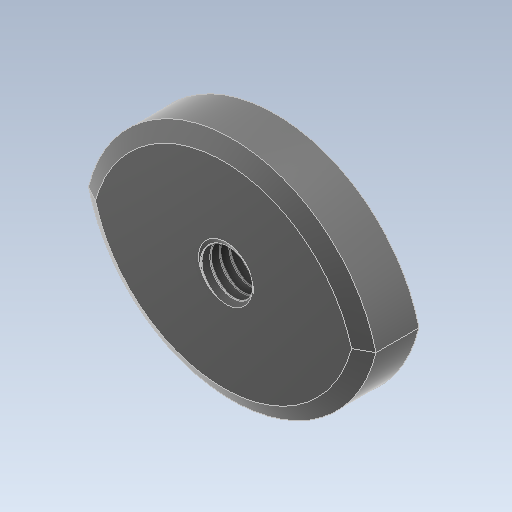
# Autodesk Inventor part: BobbinGuidePlate
Saved by Autodesk Inventor 2021 (Build 250183000, 183)
## iProperties
Created: 2020-03-09
Part Number: BobbinGuidePlate
Material: Generic
Document SubType Name: Modeling
Designer: elmar
Density: 1 g/cm^3
Appearance: Smooth - Black
Author: elmar
Autodesk Inventor part; units mm, degrees
ref_plane "YZ Plane" through (0, 0, 0) normal (1, 0, 0) x (0, 1, 0)
ref_plane "XZ Plane" through (0, 0, 0) normal (0, 1, 0) x (-1, 0, 0)
ref_plane "XY Plane" through (0, 0, 0) normal (0, 0, 1) x (1, 0, 0)
sketch "Sketch1" plane through (0, 0, 0) normal (0, 0, 1) x (1, 0, 0)
  circle A0 centre (0, 0) radius 15
  circle A1 centre (0, 0) radius 19
  arc A2 (19, 0) -> (-19, 0) centre (0, -4.5333) ccw
  arc A3 (-19, 0) -> (19, 0) centre (0, 4.5333) ccw
  line L0 (-26.6, 0) -> (26.6, 0) projected
  point P0 (0, 15)
  point P1 (0, -15)
  dimension "CarriageGuidePlateDiameter" = 30
  dimension "d70" = 38
  constraints: 6 point on circle, 4 centre point, 2 coincident, 2 point on line, 2 tangent
  measures "CarriageGuidePlateDiameter" diameter of A0
  measures "d70" diameter of A1
extrude "Extrusion1" add sketch "Sketch1" along normal blind 8 contours L0 A0 | L0 A3 A0 | A0 A2 L0 | A0 L0 | A0 L0 A2 | A3 L0 A0
sketch "Sketch2" plane through (0, 0, 0) normal (0, 0, -1) x (-1, 0, 0)
  point P0 (0, 0)
hole "Hole1" at (0, 0, 0) direction (0, 0, 1) diameter 8 end through all
thread "Thread1" size "M8x1.25" class "6H" standard "ANSI Metric M Profile" full length
sketch "Sketch8" plane through (0, 0, 0) normal (1, 0, 0) x (0, 1, 0)
  line L0 (4, 0) -> (4, 8)
  line L1 (4, 8) -> (3.0732, 8)
  line L2 (3.0732, 8) -> (3.0732, 0)
  line L3 (3.0732, 0) -> (4, 0)
  line L4 (0, -1.6) -> (0, 9.6) projected
  constraints: 8 end point
revolve "Revolution3" add sketch "Sketch8" angle 360 about axis through (0, 0, 0) along (0, 0, 1) separate body
sketch "Sketch7" plane through (0, 4, 0) normal (-1, 0, 0) x (0, 0, 1)
  line L0 (-0.7293, -0.0634) -> (-0.6251, -0.0634) construction
  line L1 (0.1041, -0.8638) -> (-0.0001, -1.0639) construction
  line L2 (-1.2501, -1.0639) -> (-1.3543, -0.8638) construction
  line L3 (-0.5209, -0.0634) -> (-0.6251, 0.1367) construction
  line L4 (-0.6251, 0.1367) -> (-0.7293, -0.0634) construction
  line L5 (-1.2501, -1.0639) -> (-1.1459, -0.8638) construction
  line L6 (-0.5209, -0.0634) -> (-0.1043, -0.8638)
  line L7 (-1.3543, -0.8638) -> (-1.1459, -0.8638) construction
  arc A0 (-1.3543, -0.8638) -> (-1.2501, -0.927) centre (-1.2501, -0.8096) ccw construction
  line L8 (0.1041, -0.8638) -> (-0.1043, -0.8638) construction
  line L9 (-1.2501, -1.0639) -> (-1.2501, -0.8638) construction
  line L10 (-0.0001, -1.0639) -> (-0.0001, -0.8638) construction
  line L11 (-0.6251, 0.1367) -> (-0.6251, -0.0002) construction
  line L12 (-1.2501, -0.927) -> (-0.0001, -0.927)
  arc A1 (-1.2501, -0.927) -> (-1.1459, -0.8638) centre (-1.2501, -0.8096) ccw
  line L13 (-0.1043, -0.8638) -> (-0.0001, -1.0639) construction
  line L14 (-1.1459, -0.8638) -> (-0.7293, -0.0634)
  line L15 (-0.0001, -0.0002) -> (-0.0001, 0.0177)
  line L16 (-0.0001, 0.0177) -> (-0.0001, -0.0002)
  line L17 (-0.0001, -0.0002) -> (0.0334, -0.0002)
  arc A2 (-0.1043, -0.8638) -> (-0.0001, -0.927) centre (-0.0001, -0.8096) ccw
  arc A3 (-0.0001, -0.927) -> (0.1041, -0.8638) centre (-0.0001, -0.8096) ccw construction
  arc A4 (-0.6251, -0.0002) -> (-0.7293, -0.0634) centre (-0.6251, -0.1176) ccw
  arc A5 (-0.5209, -0.0634) -> (-0.6251, -0.0002) centre (-0.6251, -0.1176) ccw
  line L18 (-0.6251, -0.0002) -> (-0.6251, -0.0634) construction
  line L19 (-0.6251, -0.0634) -> (-0.5209, -0.0634) construction
  dimension "d49" = 55
  dimension "d50" = 0.2001
  dimension "d51" = 0.2001
  dimension "Sketch7_ThreadOffset" = 0
  dimension "Sketch7_MajorRadius" = 0.9268
  dimension "d54" = 1.25
  dimension "Sketch7_MinorRadius" = 0
  constraints: 40 end point, 12 point on circle, 10 parallel, 8 tangent, 6 centre point, 6 collinear, 2 midpoint, 2 point on line, 1 horizontal, 1 perpendicular, 3 other
  measures "d49" angle of L6 L14
  measures "d50" distance of L3.end L0.end
  measures "d51" distance of L1.end L10.end
  measures "Sketch7_ThreadOffset" distance between parallel lines of L15 L10
  measures "Sketch7_MajorRadius" distance from line of L12 L15.start
  measures "d54" distance from line of L1.end L9
  measures "Sketch7_MinorRadius" distance edge to line of A5 L17
coil "Coil3" sketch "Sketch7" operation cut axis through (0, 0, 0) along (0, 0, 1) pitch 1.2513 turns 8.391608 hand right bodies 2
combine bodies "Combine1" operation type add bodies to combine 1 2
chamfer "Chamfer1" distance 2 angle 30 2 edges at (0, 15, 0) (0, -15, 0) measured on face at (0, 14.5, 0) measured on face at (0, -14.5, 0)
chamfer "Chamfer2" distance 2 angle 30 2 edges at (0, 15, 8) (0, -15, 8) measured on face at (0, 14.5, 8) measured on face at (0, -14.5, 8)
sketch "Sketch10" plane through (0, 4.5333, 0) normal (0, 0, -1) x (0, -1, 0)
  line L0 (4.5333, 10) -> (4.5333, -10)
  circle A0 centre (4.5333, 10) radius 1.5
  circle A1 centre (4.5333, -10) radius 1.5
  point P0 (4.5333, 0)
  point P1 (4.5333, 0)
  dimension "d77" = 20
  dimension "d78" = 3
  constraints: 3 coincident, 2 centre point, 2 end point, 1 equal radius, 1 midpoint, 1 vertical
  measures "d77" distance of L0.start L0.end
  measures "d78" diameter of A0
extrude "Extrusion2" add sketch "Sketch10" along normal blind 1 contours A1 bodies 1
hole "Hole2" at (-10, 0, 0) direction (0, 0, 1) diameter 3.2 depth 1.2 bodies 1
equation "\"d4\" = GearShaftDiameter"
equation "\"d49\" = d56"
equation "\"d50\" = 0.160083 * Sketch7_Pitch"
equation "\"d51\" = 0.160083 * Sketch7_Pitch"
equation "\"d54\" = Sketch7_Pitch"
equation "\"d20\" = 55deg"
equation "\"Sketch3_Pitch\" = 1.25"
equation "\"d38\" = 55deg"
equation "\"Sketch5_Pitch\" = 1.25"
equation "\"d56\" = 55deg"
equation "\"Sketch7_Pitch\" = 1.25"
equation "\"GearShaftDiameter\" = 8"
body "Solid1"
